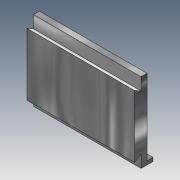
# Autodesk Inventor part: J007869 NEUROPIXELS DOVE TAIL MOUNT Rev -
Saved by Autodesk Inventor 2018.3 (Build 223284000, 284)
## iProperties
Created: 2017-01-23
Material: ALUMINUM, 6061-T651
Vendor: HHMI: JRC - ID&F
Document SubType Name: Modeling
Designer: ARNOLDJ
Density: 2.7 g/cm^3
Appearance: Metal-AL-6061 (Machined)
Description: NEUROPIXELS DOVE TAIL MOUNT
Part Number: J007869 NEUROPIXELS DOVE TAIL MOUNT Rev -
RuleStatus: InUse
AfterDocSave0: file://Part Number Cleaner
LAB/DEPT: APIG (SHARED RESOURCE)
REQUESTING SCIENTIST: BARBARTIS, BRIAN
SURFACE ROUGHNESS: 32 Ra
DESIGN DEPARTMENT: HHMI: JRC - ID&F
SPECIAL FINISH: NONE
ALTERED ITEM PART NUMBER: N/A
ALTERED ITEM VENDOR: N/A
ALTERED ITEM DESCRIPTION: N/A
Author: ARNOLDJ
Revision Number: 0
Autodesk Inventor part; units mm, degrees
ref_plane "YZ Plane" through (0, 0, 0) normal (1, 0, 0) x (0, 1, 0)
ref_plane "XZ Plane" through (0, 0, 0) normal (0, 1, 0) x (-1, 0, 0)
ref_plane "XY Plane" through (0, 0, 0) normal (0, 0, 1) x (1, 0, 0)
sketch "Sketch1" plane through (0, 0, 0) normal (0, 0, 1) x (1, 0, 0)
  line L0 (0, 4.2672) -> (0, -4.2672) projected
  line L1 (-5.7785, 0) -> (5.7785, 0) projected
  line L2 (4.1275, -3.048) -> (-4.1275, -3.048)
  line L3 (-4.1275, -3.048) -> (-4.1275, 3.048)
  line L4 (-4.1275, 3.048) -> (4.1275, 3.048)
  line L5 (4.1275, 3.048) -> (4.1275, -3.048)
  line L6 (4.1275, -3.048) -> (-4.1275, 3.048) construction
  line L7 (-4.1275, -3.048) -> (4.1275, 3.048) construction
  point P0 (0, 0)
  dimension "d0" = 8.255
  dimension "d1" = 6.096
  constraints: 12 end point, 2 midpoint, 2 parallel, 1 horizontal, 1 perpendicular
  measures "d0" distance of L3.end L4.end
  measures "d1" distance of L2.end L3.end
extrude "Extrusion1" add sketch "Sketch1" along normal blind 0.9652
sketch "Sketch2" plane through (4.1275, -3.048, 0) normal (1, 0, 0) x (0, 0, -1)
  line L0 (0, 0) -> (-0.9652, 0) projected
  line L1 (-0.9652, 0) -> (-0.9652, 6.096) projected
  line L2 (0, 6.096) -> (0, 0) projected
  line L3 (-0.4572, 0) -> (-0.4572, 0.9474)
  line L4 (-0.4572, 0.9474) -> (-0.9652, 0.6541)
  line L5 (-0.9652, 0.6541) -> (-0.9652, 0)
  line L6 (-0.9652, 0) -> (-0.4572, 0)
  line L7 (-1.1582, 3.048) -> (0.193, 3.048) projected
  point P0 (0, 3.048)
  dimension "d4" = 0.508
  dimension "d5" = 0.9474
  dimension "d6" = 60
  dimension "d15" = 0.6541
  dimension "d16" = 2.1006
  constraints: 8 end point, 2 perpendicular, 2 point on line, 1 collinear
  measures "d4" distance between parallel lines of L3 L1
  measures "d5" distance of L3.start L3.end
  measures "d6" angle of L3 L4
  measures "d15" distance from line of L0 L4.end
  measures "d16" distance from line of L3.end L7
extrude "Extrusion2" cut sketch "Sketch2" against normal blind 8.255 contours L0 L1 L4 L3
mirror "Mirror1" about plane through (0, 0, 0) normal (0, 1, 0) of "Extrusion2"
sketch "Sketch4" plane through (0, 0, 0.9652) normal (0, 0, 1) x (1, 0, 0)
  line L0 (0, 4.2672) -> (0, -4.2672) projected
  line L1 (-5.7785, 0) -> (5.7785, 0) projected
  line L2 (-4.1275, 2.3939) -> (-4.1275, -2.3939) projected
  line L3 (4.1275, -1.2192) -> (-4.1275, -1.2192)
  line L4 (-4.1275, -1.2192) -> (-4.1275, 1.2192)
  line L5 (-4.1275, 1.2192) -> (4.1275, 1.2192)
  line L6 (4.1275, 1.2192) -> (4.1275, -1.2192)
  line L7 (4.1275, -1.2192) -> (-4.1275, 1.2192) construction
  line L8 (-4.1275, -1.2192) -> (4.1275, 1.2192) construction
  point P0 (0, 0)
  dimension "d17" = 2.4384
  constraints: 12 end point, 2 midpoint, 2 parallel, 1 horizontal, 1 perpendicular, 1 point on line
  measures "d17" distance between parallel lines of L3 L5
extrude "Extrusion4" [suppressed]
sketch "Sketch5" plane through (0, 0, 0) normal (1, 0, 0) x (0, 1, 0)
  line L0 (3.048, 0) -> (-3.048, 0) projected
  line L1 (-3.048, 0) -> (-3.048, 0.4572) projected
  line L2 (3.048, 0) -> (3.048, 0.4572) projected
  line L3 (-3.048, 0) -> (-2.7686, 0)
  line L4 (-2.7686, 0) -> (-2.7686, -0.4572)
  line L5 (-2.7686, -0.4572) -> (-3.048, -0.4572)
  line L6 (-3.048, -0.4572) -> (-3.048, 0)
  line L7 (3.048, 0) -> (2.7686, 0)
  line L8 (2.7686, 0) -> (2.7686, -0.4572)
  line L9 (2.7686, -0.4572) -> (3.048, -0.4572)
  line L10 (3.048, -0.4572) -> (3.048, 0)
  point P0 (0, 0)
  dimension "d20" = 0.4572
  dimension "d21" = 5.5372
  constraints: 16 end point, 4 parallel, 2 horizontal, 2 perpendicular, 1 collinear, 1 horizontal alignment, 1 point on line
  measures "d20" distance of L5.end L0.end
  measures "d21" distance between parallel lines of L8 L4
extrude "Extrusion5" add sketch "Sketch5" against normal up to surface (8.255 mm away) from surface at 4.1275 contours L4 L5 L6 L0
body "Solid1"
